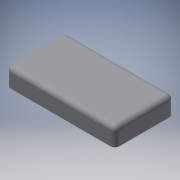
# Autodesk Inventor part: Top_Case
Saved by Autodesk Inventor 2017 (Build 210142000, 142)
## iProperties
Created: 2017-07-30
Part Number: Top_Case
Material: Generic
Document SubType Name: Modeling
Designer: Mitch
Density: 1 g/cm^3
Appearance: Default
Author: Mitch
Autodesk Inventor part; units mm, degrees
ref_plane "YZ Plane" through (0, 0, 0) normal (1, 0, 0) x (0, 1, 0)
ref_plane "XZ Plane" through (0, 0, 0) normal (0, 1, 0) x (-1, 0, 0)
ref_plane "XY Plane" through (0, 0, 0) normal (0, 0, 1) x (1, 0, 0)
sketch "Sketch1" plane through (0, 0, 0) normal (0, 1, 0) x (-1, 0, 0)
  line L0 (0, 0) -> (76.2, 0)
  line L1 (76.2, 0) -> (76.2, -41.275)
  line L2 (76.2, -41.275) -> (0, -41.275)
  line L3 (0, -41.275) -> (0, 0)
  dimension "d0" = 76.2
  dimension "d1" = 41.275
  constraints: 8 end point, 2 parallel, 1 horizontal, 1 perpendicular
  measures "d0" distance of L1.end L2.end
  measures "d1" distance of L0.end L1.end
extrude "Extrusion1" add sketch "Sketch1" along normal blind 12.7
shell "Shell1" thickness 2.54 removed faces 1 at (-25.4, 0, -13.7583)
fillet "Fillet1" radius 3.175 12 edges at (0, 6.35, 0) (0, 6.35, -41.275) (-76.2, 6.35, -41.275) (-76.2, 6.35, 0) (-76.2, 12.7, -20.6375) (-38.1, 12.7, -41.275) (0, 12.7, -20.6375) (-38.1, 12.7, 0) (-73.66, 5.08, -2.54) (-2.54, 5.08, -2.54) (-2.54, 5.08, -38.735) (-73.66, 5.08, -38.735)
sketch "Sketch2" plane through (0, 0, 0) normal (0, -1, 0) x (1, 0, 0)
  arc A0 (-73.66, -35.56) -> (-70.485, -38.735) centre (-70.485, -35.56) ccw projected
  line L0 (-5.715, -38.735) -> (-70.485, -38.735) projected
  arc A1 (-5.715, -38.735) -> (-2.54, -35.56) centre (-5.715, -35.56) ccw projected
  line L1 (-2.54, -5.715) -> (-2.54, -35.56) projected
  arc A2 (-2.54, -5.715) -> (-5.715, -2.54) centre (-5.715, -5.715) ccw projected
  line L2 (-70.485, -2.54) -> (-5.715, -2.54) projected
  arc A3 (-70.485, -2.54) -> (-73.66, -5.715) centre (-70.485, -5.715) ccw projected
  line L3 (-73.66, -35.56) -> (-73.66, -5.715) projected
  arc A4 (-1.27, -5.715) -> (-5.715, -1.27) centre (-5.715, -5.715) ccw
  line L4 (-1.27, -5.715) -> (-1.27, -35.56)
  arc A5 (-5.715, -40.005) -> (-1.27, -35.56) centre (-5.715, -35.56) ccw
  line L5 (-5.715, -40.005) -> (-70.485, -40.005)
  arc A6 (-74.93, -35.56) -> (-70.485, -40.005) centre (-70.485, -35.56) ccw
  line L6 (-74.93, -35.56) -> (-74.93, -5.715)
  arc A7 (-70.485, -1.27) -> (-74.93, -5.715) centre (-70.485, -5.715) ccw
  line L7 (-70.485, -1.27) -> (-5.715, -1.27)
  point P0 (0, 0)
  dimension "d6" = 1.27
  constraints: 8 end point, 8 point on circle, 4 centre point, 7 other
  measures "d6" distance between parallel lines of L2 L7
extrude "Extrusion2" cut sketch "Sketch2" against normal blind 2.54
sketch "Sketch3" plane through (-1.27, 0, -35.56) normal (-1, 0, 0) x (0, 0, 1)
  line L0 (11.43, 0) -> (11.43, 1.1684)
  line L1 (21.59, 0) -> (11.43, 0)
  line L2 (11.43, 0) -> (11.43, 1.1684)
  line L3 (11.43, 1.1684) -> (21.59, 1.1684)
  line L4 (21.59, 1.1684) -> (21.59, 0)
  line L5 (29.845, 0) -> (29.845, 2.54) projected
  line L6 (29.845, 0) -> (0, 0) projected
  point P0 (35.56, 0)
  dimension "d13" = 8.255
  dimension "d14" = 10.16
  dimension "d15" = 1.1684
  constraints: 10 end point, 2 parallel, 1 horizontal, 1 perpendicular
  measures "d13" distance between parallel lines of L5 L4
  measures "d14" distance between parallel lines of L0 L4
  measures "d15" distance between parallel lines of L6 L3
extrude "Extrusion3" add sketch "Sketch3" along normal blind 1.016
fillet "Fillet2" radius 0.7937 2 edges at (-2.286, 0.5842, -13.97) (-2.286, 0.5842, -24.13)
fillet "Fillet2" radius 0.508 2 edges at (-2.286, 0, -19.05) (-2.286, 1.1684, -19.05)
sketch "Sketch4" plane through (-74.93, 0, -5.715) normal (1, 0, 0) x (0, 0, -1)
  line L0 (29.845, 0) -> (0, 0) projected
  line L1 (11.43, 0) -> (11.43, 1.1684)
  line L2 (21.59, 0) -> (21.59, 1.1684)
  line L3 (21.59, 0) -> (11.43, 0)
  line L4 (11.43, 0) -> (11.43, 1.1684)
  line L5 (11.43, 1.1684) -> (21.59, 1.1684)
  line L6 (21.59, 1.1684) -> (21.59, 0)
  line L7 (29.845, 0) -> (29.845, 2.54) projected
  point P0 (-5.715, 0)
  dimension "d23" = 1.1684
  dimension "d24" = 10.16
  dimension "d25" = 8.255
  constraints: 12 end point, 2 parallel, 1 horizontal, 1 perpendicular
  measures "d23" distance between parallel lines of L0 L5
  measures "d24" distance of L1.end L5.end
  measures "d25" distance between parallel lines of L2 L7
extrude "Extrusion4" add sketch "Sketch4" along normal blind 1.016
fillet "Fillet3" radius 0.7937 2 edges at (-73.914, 0.5842, -27.305) (-73.914, 0.5842, -17.145)
fillet "Fillet3" radius 0.508 2 edges at (-73.914, 0, -22.225) (-73.914, 1.1684, -22.225)
body "Solid1"
